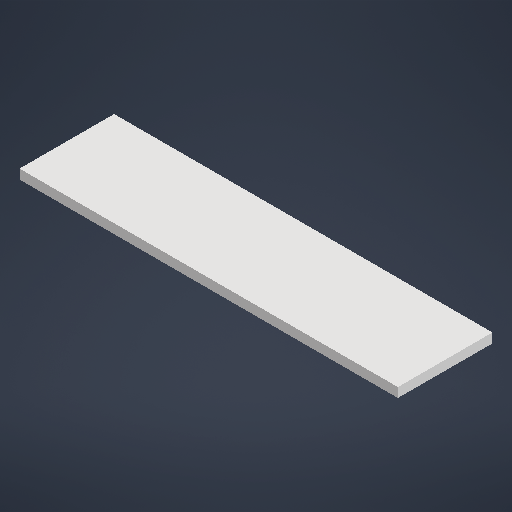
# Autodesk Inventor part: rig_connector
Saved by Autodesk Inventor 2027.1 (Build 311270010, 270A)
## iProperties
Created: 2026-09-04
Part Number: rig_connector
Material: Generic
Document SubType Name: Modeling
Designer: ajrcr
Density: 1 g/cm^3
Appearance: Default
Author: ajrcr
Autodesk Inventor part; units mm, degrees
ref_plane "YZ Plane" through (0, 0, 0) normal (1, 0, 0) x (0, 1, 0)
ref_plane "XZ Plane" through (0, 0, 0) normal (0, 1, 0) x (-1, 0, 0)
ref_plane "XY Plane" through (0, 0, 0) normal (0, 0, 1) x (1, 0, 0)
sketch "Sketch1" plane through (0, 0, 0) normal (0, 1, 0) x (-1, 0, 0)
  line L0 (-60, -15) -> (60, -15)
  line L1 (60, -15) -> (60, 15)
  line L2 (60, 15) -> (-60, 15)
  line L3 (-60, 15) -> (-60, -15)
  point P0 (0, 0)
  point P1 (60, 0)
  dimension "d0" = 120
  dimension "d1" = 30
  dimension "d2" = 60
  dimension "d3" = 15
  constraints: 8 end point, 2 parallel, 1 horizontal, 1 midpoint, 1 perpendicular
  measures "d0" distance of L2.end L1.end
  measures "d1" distance of L1.end L0.end
  measures "d2" distance of point (0, 0) point (60, 0)
  measures "d3" distance from line of L0 point (0, 0)
extrude "Extrusion1" add sketch "Sketch1" along normal blind 3
body "Solid1"
